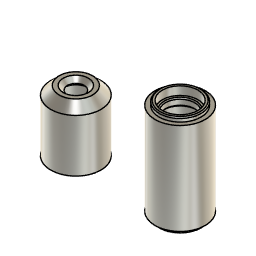
5mW Laser Pen Casing (Autodesk Fusion 360 design; units mm, degrees)
Autodesk Fusion 360 part; units mm, degrees
sketch "Sketch1" plane through (0, 0, 0) normal (0, 0, 1) x (1, 0, 0)
  circle A0 centre (0, 0) radius 4
  circle A1 centre (0, 0) radius 6
  dimension "d1" = 8
  dimension "d2" = 12
  constraint coincident A0.centre A1.centre
  constraint concentric A0 A1
  measures "d1" diameter of A0
  measures "d2" diameter of A1
extrude "Extrude1" add sketch "Sketch1" along normal blind 12.6 makes body 1
sketch "Sketch2" plane through (0, 0, 12.6) normal (0, 0, 1) x (-1, 0, 0)
  circle A0 centre (0, 0) radius 4
  circle A1 centre (0, 0) radius 6
  circle A2 centre (0, 0) radius 2
  circle A3 centre (0, 0) radius 4
  dimension "d5" = 4
  constraint concentric A0 A2
  constraint concentric A0 A3
  measures "d5" diameter of A2
extrude "Extrude2" add 1 faces at (5.2961, -0.4968, 12.6) along direction (0, 0, 1) blind 2 on bodies 1 bodies 1
extrude "Extrude3" add sketch "Sketch2" along normal blind 2 contours A0 A3 bodies 1
chamfer "Chamfer1" distance 2 angle 45 1 edges at (-5.594, -2.1697, 14.6) on bodies 1
sketch "Sketch3" plane through (0, 0, 0) normal (0, 0, 1) x (1, 0, 0)
  circle A0 centre (25, 0) radius 6
  circle A1 centre (25, 0) radius 4
  dimension "d11" = 12
  constraint concentric A0 A1
  measures "d11" diameter of A0
extrude "Extrude4" add sketch "Sketch3" along normal blind 10 separate body makes body 2
sketch "Sketch4" plane through (0, 0, 10) normal (0, 0, 1) x (-1, 0, 0)
  circle A0 centre (-25, 0) radius 4
  circle A1 centre (-25, 0) radius 6
  circle A2 centre (-25, 0) radius 2
  constraint concentric A0 A2
extrude "Extrude5" add 1 faces at (30.2961, -0.4968, 10) along direction (0, 0, 1) blind 2 on bodies 2 bodies 2
extrude "Extrude6" add sketch "Sketch4" along normal blind 2 contours A0 bodies 2
move_face "OffsetFaces1" offset -1.5 1 faces at (23.0099, 0.1991, 10.6667) on bodies 2
move_face "OffsetFaces2" offset -0.25 1 faces at (3.9801, -0.3983, 8.4) on bodies 1
move_face "OffsetFaces3" offset -0.25 1 faces at (28.9801, 0.3983, 6.6667) on bodies 2
sketch "Sketch5" plane through (0, 0, 12) normal (0, 0, 1) x (-1, 0, 0)
  circle A0 centre (-25, 0) radius 3.5
  circle A1 centre (-25, 0) radius 6
  circle A2 centre (-25, 0) radius 4
  dimension "d21" = 8
  constraint concentric A0 A2
  measures "d21" diameter of A2
extrude "Extrude7" add sketch "Sketch5" along normal blind 1 contours A1 bodies 2
extrude "Extrude8" add 1 faces at (30.3785, 0.5092, 0) along direction (0, 0, -1) blind 10 on bodies 2 bodies 2
chamfer "Chamfer2" distance 1 angle 45 1 edges at (19.406, 2.1697, -10) on bodies 2
chamfer "Chamfer5" distance 1 angle 45 1 edges at (1.8647, -0.7232, 14.6) on bodies 1
chamfer "Chamfer6" distance 1 angle 45 1 edges at (1.8647, -0.7232, 12.6) on bodies 1
move_body "Align1" bodies 2 to x (1, 0, 0) y (0, 1, 0) z (0, 0, 1) at (0, 0, 10)
sketch "Sketch7" plane through (0, 0, 0) normal (0, 0, -1) x (1, 0, 0)
  circle A0 centre (0, 0) radius 4.25
  circle A1 centre (0, 0) radius 6
  circle A2 centre (0, 0) radius 4.25
  circle A3 centre (0, 0) radius 5
  dimension "d31" = 10
  constraint coincident A0.centre A1.centre
  measures "d31" diameter of A3
sketch "Sketch8" plane through (0, 0, 23) normal (0, 0, 1) x (-1, 0, 0)
  circle A0 centre (-25, 0) radius 4
  circle A1 centre (-25, 0) radius 6
move_face "OffsetFaces4" offset -0.25 1 faces at (29.2289, 0.4232, 13.3333) on bodies 2
chamfer "Chamfer8" distance 0.5 angle 45 1 edges at (28.2631, -1.2657, 20) on bodies 2
move_face "OffsetFaces5" offset -0.25 1 faces at (21.0199, 0.3983, 22.3333) on bodies 2
chamfer "Chamfer9" distance 0.25 angle 45 1 edges at (28.2631, -1.2657, 22) on bodies 2
sketch "Sketch12" plane through (0, 0, 23) normal (0, 0, 1) x (-1, 0, 0)
  circle A0 centre (-25, 0) radius 4.25
  circle A1 centre (-25, 0) radius 6
  circle A2 centre (-25, 0) radius 4.25
  circle A3 centre (-25, 0) radius 5
  constraint concentric A0 A2
  constraint concentric A0 A3
extrude "Extrude9" add sketch "Sketch12" along normal blind 1 contours A3 bodies 2
chamfer "Chamfer10" distance 0.25 angle 45 1 edges at (29.6616, 1.8081, 24) on bodies 2
sketch "Sketch13" plane through (0, 0, 0) normal (0, 0, -1) x (1, 0, 0)
  circle A0 centre (0, 0) radius 4.25
  circle A1 centre (0, 0) radius 6
  circle A2 centre (0, 0) radius 4.25
  circle A3 centre (0, 0) radius 5.25
  dimension "d41" = 10.5
  constraint concentric A0 A2
  constraint concentric A0 A3
  measures "d41" diameter of A3
extrude "Extrude10" cut sketch "Sketch13" against normal blind 1 contours A3 bodies 1
chamfer "Chamfer11" distance 0.25 angle 45 1 edges at (-4.8947, -1.8985, 0) on bodies 1
chamfer "Chamfer12" distance 0.5 angle 45 1 edges at (-3.9624, 1.5369, 1) on bodies 1
